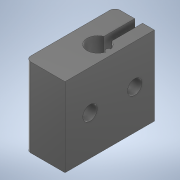
# Autodesk Inventor part: yaxissupport
Saved by Autodesk Inventor 2020.2 (Build 242310000, 310)
## iProperties
Created: 2020-07-30
Part Number: yaxissupport
Material: Generic
Document SubType Name: Modeling
Designer: JK
Density: 1 g/cm^3
Appearance: Smooth - Black
Author: JK
Autodesk Inventor part; units mm, degrees
ref_plane "YZ Plane" through (0, 0, 0) normal (1, 0, 0) x (0, 1, 0)
ref_plane "XZ Plane" through (0, 0, 0) normal (0, 1, 0) x (-1, 0, 0)
ref_plane "XY Plane" through (0, 0, 0) normal (0, 0, 1) x (1, 0, 0)
sketch "Sketch1" plane through (0, 0, 0) normal (0, 1, 0) x (-1, 0, 0)
  circle A0 centre (-1.5, 0) radius 4.1
  line L0 (-7.5, 7.5) -> (7.5, 7.5)
  line L1 (7.5, 7.5) -> (7.5, -7.5)
  line L2 (7.5, -7.5) -> (-7.5, -7.5)
  line L3 (-7.5, -7.5) -> (-7.5, 7.5)
  line L4 (-7.5, 7.5) -> (7.5, 7.5)
  line L5 (7.5, 7.5) -> (7.5, 18.5)
  line L6 (7.5, 18.5) -> (-7.5, 18.5)
  line L7 (-7.5, 18.5) -> (-7.5, 7.5)
  line L8 (7.5, -7.5) -> (-7.5, -7.5)
  line L9 (-7.5, -7.5) -> (-7.5, -15.5)
  line L10 (-7.5, -15.5) -> (7.5, -15.5)
  line L11 (7.5, -15.5) -> (7.5, -7.5)
  point P0 (-1.5, 0)
  dimension "d0" = 8.2
  dimension "d1" = 15
  dimension "d2" = 15
  dimension "d5" = 15
  dimension "d6" = 11
  dimension "d7" = 8
  dimension "d34" = 6
  constraints: 24 end point, 6 parallel, 3 horizontal, 3 perpendicular, 1 centre point, 1 collinear
  measures "d0" diameter of A0
  measures "d1" distance between parallel lines of L1 L3
  measures "d2" distance of L0.end L1.end
  measures "d5" distance of L5.end L6.end
  measures "d6" distance between parallel lines of L0 L6
  measures "d7" distance between parallel lines of L10 L2
  measures "d34" distance from line of L3 A0.centre
extrude "Extrusion1" add sketch "Sketch1" along normal blind 30
sketch "Sketch4" plane through (-7.5, 0, -15.5) normal (-1, 0, 0) x (0, 0, 1)
  circle A0 centre (7.5, 15) radius 2.75
  circle A1 centre (24.5, 15) radius 2.75
  point P0 (15.5, 0)
  dimension "d17" = 5.5
  dimension "d18" = 8
  dimension "d28" = 9
  constraints: 2 centre point, 1 equal radius, 1 horizontal alignment
  measures "d17" diameter of A0
  measures "d18" horizontal distance of point (15.5, 0) A0.centre
  measures "d28" horizontal distance of A1.centre point (15.5, 0)
extrude "Extrusion4" cut sketch "Sketch4" against normal through all
sketch "Sketch5" plane through (-7.5, 0, -15.5) normal (-1, 0, 0) x (0, 0, 1)
  circle A0 centre (7.5, 15) radius 2.75 projected
  circle A1 centre (7.5, 15) radius 5
  circle A2 centre (24.5, 15) radius 2.75 projected
  circle A3 centre (24.5, 15) radius 5
  point P0 (15.5, 0)
  dimension "d21" = 10
  constraints: 2 centre point, 2 coincident, 1 equal radius
  measures "d21" diameter of A1
extrude "Extrusion5" cut sketch "Sketch5" against normal blind 2
sketch "Sketch6" plane through (0, 30, 0) normal (0, 1, 0) x (1, 0, 0)
  line L0 (0, 2.9458) -> (3, 2.9458)
  line L1 (3, 2.9458) -> (3, 20.6423)
  line L2 (3, 20.6423) -> (0, 20.6423)
  line L3 (0, 20.6423) -> (0, 2.9458)
  circle A0 centre (1.5, 0) radius 4.1 projected
  point P0 (0, 0)
  dimension "d35" = 3
  dimension "d36" = 1.5
  constraints: 8 end point, 2 parallel, 1 horizontal, 1 perpendicular
  measures "d35" distance of L0.start L0.end
  measures "d36" distance from line of A0.centre L3
extrude "Extrusion6" cut sketch "Sketch6" against normal through all contours L3 A0 L1 L0 | L3 L2 L1 A0 picked at (1.3298, 3.3199)
sketch "Sketch7" plane through (0, 30, 0) normal (0, 1, 0) x (1, 0, 0)
  arc A0 (0, 3.8158) -> (3, 3.8158) centre (1.5, 0) ccw projected
  circle A1 centre (5.6, 0) radius 1
  point P0 (0, 0)
  point P1 (-1.3517, 2.9458)
  dimension "d31" = 2
  constraints: 1 centre point, 1 point on circle
  measures "d31" diameter of A1
extrude "Extrusion7" add sketch "Sketch7" against normal blind 9.5
fillet "Fillet1" radius 2 2 edges at (-7.5, 15, 18.5) (-7.5, 15, -15.5)
body "Solid1"
